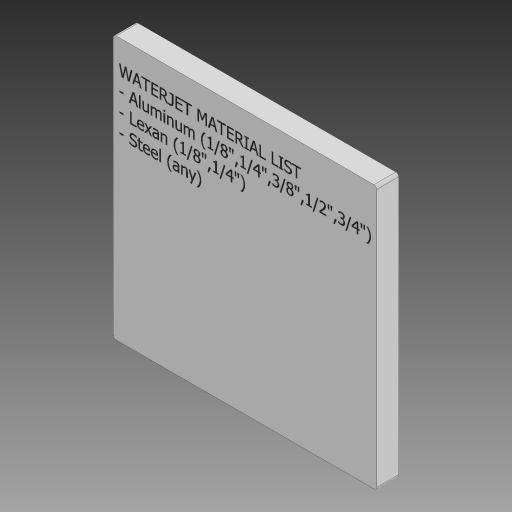
# Autodesk Inventor part: STOCK,WATERJET_MATERIALS
Saved by Autodesk Inventor 2023.4 (Build 274418000, 418)
## iProperties
Created: 2024-01-10
Part Number: STOCK,WATERJET_MATERIALS
Material: Generic
Document SubType Name: Modeling
Designer: dave.simone
Density: 1 g/cm^3
Appearance: Default
Author: dave.simone
Autodesk Inventor part; units mm, degrees
(part 1 of 2)
ref_plane "YZ Plane" through (0, 0, 0) normal (1, 0, 0) x (0, 1, 0)
ref_plane "XZ Plane" through (0, 0, 0) normal (0, 1, 0) x (-1, 0, 0)
ref_plane "XY Plane" through (0, 0, 0) normal (0, 0, 1) x (1, 0, 0)
sketch "Sketch1" plane through (0, 0, 0) normal (0, 0, 1) x (1, 0, 0)
  line L0 (-152.4, -152.4) -> (152.4, -152.4)
  line L1 (152.4, -152.4) -> (152.4, 152.4)
  line L2 (152.4, 152.4) -> (-152.4, 152.4)
  line L3 (-152.4, 152.4) -> (-152.4, -152.4)
  line L4 (-152.4, -152.4) -> (152.4, 152.4) construction
  line L5 (152.4, -152.4) -> (-152.4, 152.4) construction
  point P0 (0, 0)
  dimension "d0" = 304.8
  dimension "d1" = 304.8
  constraints: 12 end point, 2 midpoint, 2 parallel, 1 horizontal, 1 perpendicular
  measures "d0" distance of L1.end L2.end
  measures "d1" distance of L0.end L1.end
extrude "Extrusion1" add sketch "Sketch1" against normal blind 25.4
sketch "Sketch2" plane through (0, 0, 0) normal (0, 0, 1) x (1, 0, 0)
  line L0 (152.4, 152.4) -> (-152.4, 152.4) construction
  line L1 (-152.4, 152.4) -> (-152.4, -152.4) construction
  line L2 (-146.05, 127) -> (146.05, 127) construction
  line L3 (146.05, 127) -> (146.05, -127) construction
  line L4 (146.05, -127) -> (-146.05, -127) construction
  line L5 (-146.05, -127) -> (-146.05, 127) construction
  line L6 (-130.5301, 126.7736) -> (-133.7205, 114.0736)
  line L7 (-133.7205, 114.0736) -> (-135.6142, 114.0736)
  line L8 (-135.6142, 114.0736) -> (-138.1974, 124.6123)
  line L9 (-138.1974, 124.6123) -> (-140.7086, 114.0736)
  line L10 (-140.7086, 114.0736) -> (-142.5817, 114.0736)
  line L11 (-142.5817, 114.0736) -> (-145.8236, 126.7736)
  line L12 (-145.8236, 126.7736) -> (-144.0843, 126.7736)
  line L13 (-144.0843, 126.7736) -> (-141.5319, 116.2451)
  line L14 (-141.5319, 116.2451) -> (-139.0002, 126.7736)
  line L15 (-139.0002, 126.7736) -> (-137.2814, 126.7736)
  line L16 (-137.2814, 126.7736) -> (-134.7291, 116.1216)
  line L17 (-134.7291, 116.1216) -> (-132.187, 126.7736)
  line L18 (-132.187, 126.7736) -> (-130.5301, 126.7736)
  line L19 (-130.386, 114.0736) -> (-126.1046, 126.7736)
  line L20 (-126.1046, 126.7736) -> (-124.0257, 126.7736)
  line L21 (-124.0257, 126.7736) -> (-119.7443, 114.0736)
  line L22 (-119.7443, 114.0736) -> (-121.5248, 114.0736)
  line L23 (-121.5248, 114.0736) -> (-122.6775, 117.6242)
  line L24 (-122.6775, 117.6242) -> (-127.5249, 117.6242)
  line L25 (-127.5249, 117.6242) -> (-128.6776, 114.0736)
  line L26 (-128.6776, 114.0736) -> (-130.386, 114.0736)
  line L27 (-123.1406, 119.0651) -> (-125.1063, 125.0446)
  line L28 (-125.1063, 125.0446) -> (-127.0618, 119.0651)
  line L29 (-127.0618, 119.0651) -> (-123.1406, 119.0651)
  line L30 (-115.5762, 114.0736) -> (-115.5762, 125.271)
  line L31 (-115.5762, 125.271) -> (-119.837, 125.271)
  line L32 (-119.837, 125.271) -> (-119.837, 126.7736)
  line L33 (-119.837, 126.7736) -> (-109.6276, 126.7736)
  line L34 (-109.6276, 126.7736) -> (-109.6276, 125.271)
  line L35 (-109.6276, 125.271) -> (-113.8883, 125.271)
  line L36 (-113.8883, 125.271) -> (-113.8883, 114.0736)
  line L37 (-113.8883, 114.0736) -> (-115.5762, 114.0736)
  line L38 (-108.3411, 114.0736) -> (-108.3411, 126.7736)
  line L39 (-108.3411, 126.7736) -> (-100.3959, 126.7736)
  line L40 (-100.3959, 126.7736) -> (-100.3959, 125.271)
  line L41 (-100.3959, 125.271) -> (-106.6532, 125.271)
  line L42 (-106.6532, 125.271) -> (-106.6532, 121.7924)
  line L43 (-106.6532, 121.7924) -> (-100.8178, 121.7924)
  line L44 (-100.8178, 121.7924) -> (-100.8178, 120.2898)
  line L45 (-100.8178, 120.2898) -> (-106.6532, 120.2898)
  line L46 (-106.6532, 120.2898) -> (-106.6532, 115.5762)
  line L47 (-106.6532, 115.5762) -> (-100.3959, 115.5762)
  line L48 (-100.3959, 115.5762) -> (-100.3959, 114.0736)
  line L49 (-100.3959, 114.0736) -> (-108.3411, 114.0736)
  line L50 (-88.7147, 114.0736) -> (-90.9069, 114.0736)
  line L51 (-90.9069, 114.0736) -> (-94.9207, 119.1268)
  line L52 (-94.9207, 119.1268) -> (-96.8555, 119.1268)
  line L53 (-96.8555, 119.1268) -> (-96.8555, 114.0736)
  line L54 (-96.8555, 114.0736) -> (-98.5434, 114.0736)
  line L55 (-98.5434, 114.0736) -> (-98.5434, 126.7736)
  line L56 (-98.5434, 126.7736) -> (-95.2706, 126.7736)
  spline S0 degree 2 poles (-95.2706, 126.7736) (-94.1797, 126.7736) (-92.7079, 126.5369) (-92.039, 126.1046) knots 0 0 0 1 2 2 2
  spline S1 degree 2 poles (-92.039, 126.1046) (-91.37, 125.6724) (-90.5981, 124.3241) (-90.5981, 123.3259) knots 0 0 0 1 2 2 2
  spline S2 degree 2 poles (-90.5981, 123.3259) (-90.5981, 121.9365) (-92.0184, 120.0531) (-93.2328, 119.6002) knots 0 0 0 1 2 2 2
  line L57 (-93.2328, 119.6002) -> (-88.7147, 114.0736)
  spline S3 degree 2 poles (-92.358, 123.1921) (-92.358, 123.7478) (-92.7491, 124.602) (-93.1608, 124.8799) knots 0 0 0 1 2 2 2
  spline S4 degree 2 poles (-93.1608, 124.8799) (-93.521, 125.1166) (-94.4781, 125.3122) (-95.178, 125.3122) knots 0 0 0 1 2 2 2
  line L58 (-95.178, 125.3122) -> (-96.8555, 125.3122)
  line L59 (-96.8555, 125.3122) -> (-96.8555, 120.5368)
  line L60 (-96.8555, 120.5368) -> (-95.3735, 120.5368)
  spline S5 degree 2 poles (-95.3735, 120.5368) (-94.6428, 120.5368) (-93.4798, 120.7941) (-93.0784, 121.1955) knots 0 0 0 1 2 2 2
  spline S6 degree 2 poles (-93.0784, 121.1955) (-92.7079, 121.5454) (-92.358, 122.5334) (-92.358, 123.1921) knots 0 0 0 1 2 2 2
  spline S7 degree 2 poles (-82.9205, 117.3772) (-82.9205, 115.71) (-84.9583, 113.8986) (-86.677, 113.8986) knots 0 0 0 1 2 2 2
  spline S8 degree 2 poles (-86.677, 113.8986) (-87.0887, 113.8986) (-88.4575, 114.0427) (-88.9206, 114.1456) knots 0 0 0 1 2 2 2
  line L61 (-88.9206, 114.1456) -> (-88.9206, 115.7717)
  line L62 (-88.9206, 115.7717) -> (-88.828, 115.7717)
  spline S9 degree 2 poles (-88.828, 115.7717) (-88.478, 115.6482) (-87.4386, 115.36) (-86.9034, 115.36) knots 0 0 0 1 2 2 2
  spline S10 degree 2 poles (-86.9034, 115.36) (-86.1212, 115.36) (-85.1847, 115.7203) (-84.9686, 116.0496) knots 0 0 0 1 2 2 2
  spline S11 degree 2 poles (-84.9686, 116.0496) (-84.7318, 116.3892) (-84.6083, 117.3772) (-84.6083, 118.0256) knots 0 0 0 1 2 2 2
  line L63 (-84.6083, 118.0256) -> (-84.6083, 125.4254)
  line L64 (-84.6083, 125.4254) -> (-87.2945, 125.4254)
  line L65 (-87.2945, 125.4254) -> (-87.2945, 126.7736)
  line L66 (-87.2945, 126.7736) -> (-82.9205, 126.7736)
  line L67 (-82.9205, 126.7736) -> (-82.9205, 117.3772)
  line L68 (-80.4299, 114.0736) -> (-80.4299, 126.7736)
  line L69 (-80.4299, 126.7736) -> (-72.4847, 126.7736)
  line L70 (-72.4847, 126.7736) -> (-72.4847, 125.271)
  line L71 (-72.4847, 125.271) -> (-78.7421, 125.271)
  line L72 (-78.7421, 125.271) -> (-78.7421, 121.7924)
  line L73 (-78.7421, 121.7924) -> (-72.9066, 121.7924)
  line L74 (-72.9066, 121.7924) -> (-72.9066, 120.2898)
  line L75 (-72.9066, 120.2898) -> (-78.7421, 120.2898)
  line L76 (-78.7421, 120.2898) -> (-78.7421, 115.5762)
  line L77 (-78.7421, 115.5762) -> (-72.4847, 115.5762)
  line L78 (-72.4847, 115.5762) -> (-72.4847, 114.0736)
  line L79 (-72.4847, 114.0736) -> (-80.4299, 114.0736)
  line L80 (-67.6682, 114.0736) -> (-67.6682, 125.271)
  line L81 (-67.6682, 125.271) -> (-71.9289, 125.271)
  line L82 (-71.9289, 125.271) -> (-71.9289, 126.7736)
  line L83 (-71.9289, 126.7736) -> (-61.7195, 126.7736)
  line L84 (-61.7195, 126.7736) -> (-61.7195, 125.271)
  line L85 (-61.7195, 125.271) -> (-65.9803, 125.271)
  line L86 (-65.9803, 125.271) -> (-65.9803, 114.0736)
  line L87 (-65.9803, 114.0736) -> (-67.6682, 114.0736)
  line L88 (-44.0898, 114.0736) -> (-45.7776, 114.0736)
  line L89 (-45.7776, 114.0736) -> (-45.7776, 125.0137)
  line L90 (-45.7776, 125.0137) -> (-49.0916, 117.5728)
  line L91 (-49.0916, 117.5728) -> (-50.1207, 117.5728)
  line L92 (-50.1207, 117.5728) -> (-53.4038, 125.0137)
  line L93 (-53.4038, 125.0137) -> (-53.4038, 114.0736)
  line L94 (-53.4038, 114.0736) -> (-54.9784, 114.0736)
  line L95 (-54.9784, 114.0736) -> (-54.9784, 126.7736)
  line L96 (-54.9784, 126.7736) -> (-52.6731, 126.7736)
  line L97 (-52.6731, 126.7736) -> (-49.5032, 119.7032)
  line L98 (-49.5032, 119.7032) -> (-46.4363, 126.7736)
  line L99 (-46.4363, 126.7736) -> (-44.0898, 126.7736)
  line L100 (-44.0898, 126.7736) -> (-44.0898, 114.0736)
  line L101 (-42.8857, 114.0736) -> (-38.6043, 126.7736)
  line L102 (-38.6043, 126.7736) -> (-36.5254, 126.7736)
  line L103 (-36.5254, 126.7736) -> (-32.244, 114.0736)
  line L104 (-32.244, 114.0736) -> (-34.0245, 114.0736)
  line L105 (-34.0245, 114.0736) -> (-35.1771, 117.6242)
  line L106 (-35.1771, 117.6242) -> (-40.0246, 117.6242)
  line L107 (-40.0246, 117.6242) -> (-41.1772, 114.0736)
  line L108 (-41.1772, 114.0736) -> (-42.8857, 114.0736)
  line L109 (-35.6403, 119.0651) -> (-37.606, 125.0446)
  line L110 (-37.606, 125.0446) -> (-39.5614, 119.0651)
  line L111 (-39.5614, 119.0651) -> (-35.6403, 119.0651)
  line L112 (-28.0759, 114.0736) -> (-28.0759, 125.271)
  line L113 (-28.0759, 125.271) -> (-32.3366, 125.271)
  line L114 (-32.3366, 125.271) -> (-32.3366, 126.7736)
  line L115 (-32.3366, 126.7736) -> (-22.1272, 126.7736)
  line L116 (-22.1272, 126.7736) -> (-22.1272, 125.271)
  line L117 (-22.1272, 125.271) -> (-26.388, 125.271)
  line L118 (-26.388, 125.271) -> (-26.388, 114.0736)
  line L119 (-26.388, 114.0736) -> (-28.0759, 114.0736)
  line L120 (-20.8408, 114.0736) -> (-20.8408, 126.7736)
  line L121 (-20.8408, 126.7736) -> (-12.8955, 126.7736)
  line L122 (-12.8955, 126.7736) -> (-12.8955, 125.271)
  line L123 (-12.8955, 125.271) -> (-19.1529, 125.271)
  line L124 (-19.1529, 125.271) -> (-19.1529, 121.7924)
  line L125 (-19.1529, 121.7924) -> (-13.3175, 121.7924)
  line L126 (-13.3175, 121.7924) -> (-13.3175, 120.2898)
  line L127 (-13.3175, 120.2898) -> (-19.1529, 120.2898)
  line L128 (-19.1529, 120.2898) -> (-19.1529, 115.5762)
  line L129 (-19.1529, 115.5762) -> (-12.8955, 115.5762)
  line L130 (-12.8955, 115.5762) -> (-12.8955, 114.0736)
  line L131 (-12.8955, 114.0736) -> (-20.8408, 114.0736)
  line L132 (-1.2144, 114.0736) -> (-3.4066, 114.0736)
  line L133 (-3.4066, 114.0736) -> (-7.4203, 119.1268)
  line L134 (-7.4203, 119.1268) -> (-9.3552, 119.1268)
  line L135 (-9.3552, 119.1268) -> (-9.3552, 114.0736)
  line L136 (-9.3552, 114.0736) -> (-11.043, 114.0736)
  line L137 (-11.043, 114.0736) -> (-11.043, 126.7736)
  line L138 (-11.043, 126.7736) -> (-7.7703, 126.7736)
  spline S12 degree 2 poles (-7.7703, 126.7736) (-6.6793, 126.7736) (-5.2076, 126.5369) (-4.5387, 126.1046) knots 0 0 0 1 2 2 2
  spline S13 degree 2 poles (-4.5387, 126.1046) (-3.8697, 125.6724) (-3.0978, 124.3241) (-3.0978, 123.3259) knots 0 0 0 1 2 2 2
  spline S14 degree 2 poles (-3.0978, 123.3259) (-3.0978, 121.9365) (-4.5181, 120.0531) (-5.7325, 119.6002) knots 0 0 0 1 2 2 2
  line L139 (-5.7325, 119.6002) -> (-1.2144, 114.0736)
  spline S15 degree 2 poles (-4.8577, 123.1921) (-4.8577, 123.7478) (-5.2488, 124.602) (-5.6605, 124.8799) knots 0 0 0 1 2 2 2
  spline S16 degree 2 poles (-5.6605, 124.8799) (-6.0207, 125.1166) (-6.9778, 125.3122) (-7.6776, 125.3122) knots 0 0 0 1 2 2 2
  line L140 (-7.6776, 125.3122) -> (-9.3552, 125.3122)
  line L141 (-9.3552, 125.3122) -> (-9.3552, 120.5368)
  line L142 (-9.3552, 120.5368) -> (-7.8732, 120.5368)
  spline S17 degree 2 poles (-7.8732, 120.5368) (-7.1425, 120.5368) (-5.9795, 120.7941) (-5.5781, 121.1955) knots 0 0 0 1 2 2 2
  spline S18 degree 2 poles (-5.5781, 121.1955) (-5.2076, 121.5454) (-4.8577, 122.5334) (-4.8577, 123.1921) knots 0 0 0 1 2 2 2
  line L143 (4.2196, 114.0736) -> (-0.6998, 114.0736)
  line L144 (-0.6998, 114.0736) -> (-0.6998, 115.3703)
  line L145 (-0.6998, 115.3703) -> (0.916, 115.3703)
  line L146 (0.916, 115.3703) -> (0.916, 125.4768)
  line L147 (0.916, 125.4768) -> (-0.6998, 125.4768)
  line L148 (-0.6998, 125.4768) -> (-0.6998, 126.7736)
  line L149 (-0.6998, 126.7736) -> (4.2196, 126.7736)
  line L150 (4.2196, 126.7736) -> (4.2196, 125.4768)
  line L151 (4.2196, 125.4768) -> (2.6038, 125.4768)
  line L152 (2.6038, 125.4768) -> (2.6038, 115.3703)
  line L153 (2.6038, 115.3703) -> (4.2196, 115.3703)
  line L154 (4.2196, 115.3703) -> (4.2196, 114.0736)
  line L155 (4.94, 114.0736) -> (9.2214, 126.7736)
  line L156 (9.2214, 126.7736) -> (11.3003, 126.7736)
  line L157 (11.3003, 126.7736) -> (15.5817, 114.0736)
  line L158 (15.5817, 114.0736) -> (13.8012, 114.0736)
  line L159 (13.8012, 114.0736) -> (12.6485, 117.6242)
  line L160 (12.6485, 117.6242) -> (7.8011, 117.6242)
  line L161 (7.8011, 117.6242) -> (6.6485, 114.0736)
  line L162 (6.6485, 114.0736) -> (4.94, 114.0736)
  line L163 (12.1854, 119.0651) -> (10.2197, 125.0446)
  line L164 (10.2197, 125.0446) -> (8.2643, 119.0651)
  line L165 (8.2643, 119.0651) -> (12.1854, 119.0651)
  line L166 (24.1444, 114.0736) -> (16.7858, 114.0736)
  line L167 (16.7858, 114.0736) -> (16.7858, 126.7736)
  line L168 (16.7858, 126.7736) -> (18.4737, 126.7736)
  line L169 (18.4737, 126.7736) -> (18.4737, 115.5762)
  line L170 (18.4737, 115.5762) -> (24.1444, 115.5762)
  line L171 (24.1444, 115.5762) -> (24.1444, 114.0736)
  line L172 (38.2852, 114.0736) -> (30.9267, 114.0736)
  line L173 (30.9267, 114.0736) -> (30.9267, 126.7736)
  line L174 (30.9267, 126.7736) -> (32.6145, 126.7736)
  line L175 (32.6145, 126.7736) -> (32.6145, 115.5762)
  line L176 (32.6145, 115.5762) -> (38.2852, 115.5762)
  line L177 (38.2852, 115.5762) -> (38.2852, 114.0736)
  line L178 (44.0383, 114.0736) -> (39.1189, 114.0736)
  line L179 (39.1189, 114.0736) -> (39.1189, 115.3703)
  line L180 (39.1189, 115.3703) -> (40.7347, 115.3703)
  line L181 (40.7347, 115.3703) -> (40.7347, 125.4768)
  line L182 (40.7347, 125.4768) -> (39.1189, 125.4768)
  line L183 (39.1189, 125.4768) -> (39.1189, 126.7736)
  line L184 (39.1189, 126.7736) -> (44.0383, 126.7736)
  line L185 (44.0383, 126.7736) -> (44.0383, 125.4768)
  line L186 (44.0383, 125.4768) -> (42.4225, 125.4768)
  line L187 (42.4225, 125.4768) -> (42.4225, 115.3703)
  line L188 (42.4225, 115.3703) -> (44.0383, 115.3703)
  line L189 (44.0383, 115.3703) -> (44.0383, 114.0736)
  spline S19 degree 2 poles (49.6679, 113.8472) (48.2888, 113.8472) (46.354, 114.4235) (45.4998, 114.8352) knots 0 0 0 1 2 2 2
  line L190 (45.4998, 114.8352) -> (45.4998, 116.9553)
  line L191 (45.4998, 116.9553) -> (45.6233, 116.9553)
  spline S20 degree 2 poles (45.6233, 116.9553) (46.4569, 116.1731) (48.5667, 115.3086) (49.5444, 115.3086) knots 0 0 0 1 2 2 2
  spline S21 degree 2 poles (49.5444, 115.3086) (50.9441, 115.3086) (52.3746, 116.4716) (52.3746, 117.4287) knots 0 0 0 1 2 2 2
  spline S22 degree 2 poles (52.3746, 117.4287) (52.3746, 118.1903) (51.6233, 119.1371) (50.8103, 119.3738) knots 0 0 0 1 2 2 2
  spline S23 degree 2 poles (50.8103, 119.3738) (50.2237, 119.5385) (49.2459, 119.7649) (48.5152, 119.9502) knots 0 0 0 1 2 2 2
  spline S24 degree 2 poles (48.5152, 119.9502) (47.8566, 120.1251) (46.8171, 120.65) (46.4157, 121.072) knots 0 0 0 1 2 2 2
  spline S25 degree 2 poles (46.4157, 121.072) (46.0246, 121.4939) (45.5924, 122.626) (45.5924, 123.367) knots 0 0 0 1 2 2 2
  spline S26 degree 2 poles (45.5924, 123.367) (45.5924, 124.9108) (48.0006, 127) (49.8634, 127) knots 0 0 0 1 2 2 2
  spline S27 degree 2 poles (49.8634, 127) (50.9338, 127) (52.8275, 126.578) (53.6405, 126.1767) knots 0 0 0 1 2 2 2
  line L192 (53.6405, 126.1767) -> (53.6405, 124.1595)
  line L193 (53.6405, 124.1595) -> (53.517, 124.1595)
  spline S28 degree 2 poles (53.517, 124.1595) (52.9098, 124.7152) (51.0161, 125.5386) (49.9767, 125.5386) knots 0 0 0 1 2 2 2
  spline S29 degree 2 poles (49.9767, 125.5386) (48.8034, 125.5386) (47.3523, 124.4374) (47.3523, 123.542) knots 0 0 0 1 2 2 2
  spline S30 degree 2 poles (47.3523, 123.542) (47.3523, 122.7392) (48.2065, 121.7821) (49.0092, 121.566) knots 0 0 0 1 2 2 2
  spline S31 degree 2 poles (49.0092, 121.566) (49.5444, 121.4219) (51.0985, 121.0514) (51.613, 120.897) knots 0 0 0 1 2 2 2
  spline S32 degree 2 poles (51.613, 120.897) (52.9201, 120.4956) (54.1345, 118.8798) (54.1345, 117.6963) knots 0 0 0 1 2 2 2
  spline S33 degree 2 poles (54.1345, 117.6963) (54.1345, 116.945) (53.5273, 115.5041) (52.9818, 114.9998) knots 0 0 0 1 2 2 2
  spline S34 degree 2 poles (52.9818, 114.9998) (52.3746, 114.4441) (50.8309, 113.8472) (49.6679, 113.8472) knots 0 0 0 1 2 2 2
  line L194 (58.8173, 114.0736) -> (58.8173, 125.271)
  line L195 (58.8173, 125.271) -> (54.5565, 125.271)
  line L196 (54.5565, 125.271) -> (54.5565, 126.7736)
  line L197 (54.5565, 126.7736) -> (64.7659, 126.7736)
  line L198 (64.7659, 126.7736) -> (64.7659, 125.271)
  line L199 (64.7659, 125.271) -> (60.5051, 125.271)
  line L200 (60.5051, 125.271) -> (60.5051, 114.0736)
  line L201 (60.5051, 114.0736) -> (58.8173, 114.0736)
  line L202 (-140.4719, 97.949) -> (-145.2781, 97.949)
  line L203 (-145.2781, 97.949) -> (-145.2781, 99.4928)
  line L204 (-145.2781, 99.4928) -> (-140.4719, 99.4928)
  line L205 (-140.4719, 99.4928) -> (-140.4719, 97.949)
  line L206 (-134.338, 93.1634) -> (-130.0566, 105.8634)
  line L207 (-130.0566, 105.8634) -> (-127.9777, 105.8634)
  line L208 (-127.9777, 105.8634) -> (-123.6964, 93.1634)
  line L209 (-123.6964, 93.1634) -> (-125.4768, 93.1634)
  line L210 (-125.4768, 93.1634) -> (-126.6295, 96.714)
  line L211 (-126.6295, 96.714) -> (-131.4769, 96.714)
  line L212 (-131.4769, 96.714) -> (-132.6296, 93.1634)
  line L213 (-132.6296, 93.1634) -> (-134.338, 93.1634)
  line L214 (-127.0926, 98.1549) -> (-129.0583, 104.1344)
  line L215 (-129.0583, 104.1344) -> (-131.0138, 98.1549)
  line L216 (-131.0138, 98.1549) -> (-127.0926, 98.1549)
  line L217 (-120.9793, 93.1634) -> (-122.5848, 93.1634)
  line L218 (-122.5848, 93.1634) -> (-122.5848, 106.4294)
  line L219 (-122.5848, 106.4294) -> (-120.9793, 106.4294)
  line L220 (-120.9793, 106.4294) -> (-120.9793, 93.1634)
  line L221 (-111.2125, 93.1634) -> (-112.818, 93.1634)
  line L222 (-112.818, 93.1634) -> (-112.818, 94.2131)
  spline S35 degree 2 poles (-112.818, 94.2131) (-113.559, 93.5647) (-114.8866, 92.8958) (-115.71, 92.8958) knots 0 0 0 1 2 2 2
  spline S36 degree 2 poles (-115.71, 92.8958) (-116.3275, 92.8958) (-117.4287, 93.3075) (-117.8301, 93.75) knots 0 0 0 1 2 2 2
  spline S37 degree 2 poles (-117.8301, 93.75) (-118.2417, 94.1925) (-118.6946, 95.5408) (-118.6946, 96.5082) knots 0 0 0 1 2 2 2
  line L223 (-118.6946, 96.5082) -> (-118.6946, 102.6935)
  line L224 (-118.6946, 102.6935) -> (-117.0891, 102.6935)
  line L225 (-117.0891, 102.6935) -> (-117.0891, 97.2595)
  spline S38 degree 2 poles (-117.0891, 97.2595) (-117.0891, 96.4979) (-116.9759, 95.4996) (-116.7803, 95.1291) knots 0 0 0 1 2 2 2
  spline S39 degree 2 poles (-116.7803, 95.1291) (-116.5848, 94.7586) (-115.9158, 94.419) (-115.288, 94.419) knots 0 0 0 1 2 2 2
  spline S40 degree 2 poles (-115.288, 94.419) (-114.7014, 94.419) (-113.3737, 95.0879) (-112.818, 95.5716) knots 0 0 0 1 2 2 2
  line L226 (-112.818, 95.5716) -> (-112.818, 102.6935)
  line L227 (-112.818, 102.6935) -> (-111.2125, 102.6935)
  line L228 (-111.2125, 102.6935) -> (-111.2125, 93.1634)
  line L229 (-98.0802, 93.1634) -> (-98.0802, 98.6797)
  spline S41 degree 2 poles (-98.0802, 98.6797) (-98.0802, 99.3384) (-98.1831, 100.4602) (-98.3478, 100.769) knots 0 0 0 1 2 2 2
  spline S42 degree 2 poles (-98.3478, 100.769) (-98.5125, 101.1086) (-99.1403, 101.4379) (-99.6857, 101.4379) knots 0 0 0 1 2 2 2
  spline S43 degree 2 poles (-99.6857, 101.4379) (-100.1797, 101.4379) (-101.3118, 100.8307) (-101.9088, 100.2544) knots 0 0 0 1 2 2 2
  spline S44 degree 2 poles (-101.9088, 100.2544) (-101.8985, 100.1103) (-101.8779, 99.7089) (-101.8779, 99.4413) knots 0 0 0 1 2 2 2
  line L230 (-101.8779, 99.4413) -> (-101.8779, 93.1634)
  line L231 (-101.8779, 93.1634) -> (-103.4834, 93.1634)
  line L232 (-103.4834, 93.1634) -> (-103.4834, 98.6797)
  spline S45 degree 2 poles (-103.4834, 98.6797) (-103.4834, 99.3384) (-103.5863, 100.4602) (-103.751, 100.769) knots 0 0 0 1 2 2 2
  spline S46 degree 2 poles (-103.751, 100.769) (-103.9156, 101.1086) (-104.5434, 101.4379) (-105.0889, 101.4379) knots 0 0 0 1 2 2 2
  spline S47 degree 2 poles (-105.0889, 101.4379) (-105.6035, 101.4379) (-106.7459, 100.7895) (-107.281, 100.2852) knots 0 0 0 1 2 2 2
  line L233 (-107.281, 100.2852) -> (-107.281, 93.1634)
  line L234 (-107.281, 93.1634) -> (-108.8865, 93.1634)
  line L235 (-108.8865, 93.1634) -> (-108.8865, 102.6935)
  line L236 (-108.8865, 102.6935) -> (-107.281, 102.6935)
  line L237 (-107.281, 102.6935) -> (-107.281, 101.6438)
  spline S48 degree 2 poles (-107.281, 101.6438) (-106.6532, 102.2716) (-105.4182, 102.9611) (-104.6772, 102.9611) knots 0 0 0 1 2 2 2
  spline S49 degree 2 poles (-104.6772, 102.9611) (-103.8333, 102.9611) (-102.5263, 102.1892) (-102.1866, 101.3144) knots 0 0 0 1 2 2 2
  spline S50 degree 2 poles (-102.1866, 101.3144) (-101.4559, 102.1275) (-100.0768, 102.9611) (-99.2741, 102.9611) knots 0 0 0 1 2 2 2
  spline S51 degree 2 poles (-99.2741, 102.9611) (-98.6566, 102.9611) (-97.648, 102.5803) (-97.2775, 102.1481) knots 0 0 0 1 2 2 2
  spline S52 degree 2 poles (-97.2775, 102.1481) (-96.8967, 101.7158) (-96.4747, 100.419) (-96.4747, 99.4413) knots 0 0 0 1 2 2 2
  line L238 (-96.4747, 99.4413) -> (-96.4747, 93.1634)
  line L239 (-96.4747, 93.1634) -> (-98.0802, 93.1634)
  line L240 (-92.5844, 93.1634) -> (-94.19, 93.1634)
  line L241 (-94.19, 93.1634) -> (-94.19, 102.6935)
  line L242 (-94.19, 102.6935) -> (-92.5844, 102.6935)
  line L243 (-92.5844, 102.6935) -> (-92.5844, 93.1634)
  line L244 (-92.4712, 104.2784) -> (-94.2929, 104.2784)
  line L245 (-94.2929, 104.2784) -> (-94.2929, 105.9457)
  line L246 (-94.2929, 105.9457) -> (-92.4712, 105.9457)
  line L247 (-92.4712, 105.9457) -> (-92.4712, 104.2784)
  line L248 (-82.7455, 93.1634) -> (-84.3511, 93.1634)
  line L249 (-84.3511, 93.1634) -> (-84.3511, 98.5974)
  spline S53 degree 2 poles (-84.3511, 98.5974) (-84.3511, 99.2561) (-84.4746, 100.3882) (-84.6598, 100.7278) knots 0 0 0 1 2 2 2
  spline S54 degree 2 poles (-84.6598, 100.7278) (-84.8553, 101.088) (-85.5552, 101.4379) (-86.1521, 101.4379) knots 0 0 0 1 2 2 2
  spline S55 degree 2 poles (-86.1521, 101.4379) (-86.749, 101.4379) (-88.0149, 100.7998) (-88.6221, 100.2852) knots 0 0 0 1 2 2 2
  line L250 (-88.6221, 100.2852) -> (-88.6221, 93.1634)
  line L251 (-88.6221, 93.1634) -> (-90.2276, 93.1634)
  line L252 (-90.2276, 93.1634) -> (-90.2276, 102.6935)
  line L253 (-90.2276, 102.6935) -> (-88.6221, 102.6935)
  line L254 (-88.6221, 102.6935) -> (-88.6221, 101.6335)
  spline S56 degree 2 poles (-88.6221, 101.6335) (-87.9017, 102.2818) (-86.5123, 102.9611) (-85.7301, 102.9611) knots 0 0 0 1 2 2 2
  spline S57 degree 2 poles (-85.7301, 102.9611) (-84.3305, 102.9611) (-82.7455, 101.1086) (-82.7455, 99.3487) knots 0 0 0 1 2 2 2
  line L255 (-82.7455, 99.3487) -> (-82.7455, 93.1634)
  line L256 (-73.0816, 93.1634) -> (-74.6871, 93.1634)
  line L257 (-74.6871, 93.1634) -> (-74.6871, 94.2131)
  spline S58 degree 2 poles (-74.6871, 94.2131) (-75.4281, 93.5647) (-76.7558, 92.8958) (-77.5791, 92.8958) knots 0 0 0 1 2 2 2
  spline S59 degree 2 poles (-77.5791, 92.8958) (-78.1966, 92.8958) (-79.2978, 93.3075) (-79.6992, 93.75) knots 0 0 0 1 2 2 2
  spline S60 degree 2 poles (-79.6992, 93.75) (-80.1109, 94.1925) (-80.5637, 95.5408) (-80.5637, 96.5082) knots 0 0 0 1 2 2 2
  line L258 (-80.5637, 96.5082) -> (-80.5637, 102.6935)
  line L259 (-80.5637, 102.6935) -> (-78.9582, 102.6935)
  line L260 (-78.9582, 102.6935) -> (-78.9582, 97.2595)
  spline S61 degree 2 poles (-78.9582, 97.2595) (-78.9582, 96.4979) (-78.845, 95.4996) (-78.6494, 95.1291) knots 0 0 0 1 2 2 2
  spline S62 degree 2 poles (-78.6494, 95.1291) (-78.4539, 94.7586) (-77.7849, 94.419) (-77.1571, 94.419) knots 0 0 0 1 2 2 2
  spline S63 degree 2 poles (-77.1571, 94.419) (-76.5705, 94.419) (-75.2429, 95.0879) (-74.6871, 95.5716) knots 0 0 0 1 2 2 2
  line L261 (-74.6871, 95.5716) -> (-74.6871, 102.6935)
  line L262 (-74.6871, 102.6935) -> (-73.0816, 102.6935)
  line L263 (-73.0816, 102.6935) -> (-73.0816, 93.1634)
  line L264 (-59.9494, 93.1634) -> (-59.9494, 98.6797)
  spline S64 degree 2 poles (-59.9494, 98.6797) (-59.9494, 99.3384) (-60.0523, 100.4602) (-60.2169, 100.769) knots 0 0 0 1 2 2 2
  spline S65 degree 2 poles (-60.2169, 100.769) (-60.3816, 101.1086) (-61.0094, 101.4379) (-61.5549, 101.4379) knots 0 0 0 1 2 2 2
  spline S66 degree 2 poles (-61.5549, 101.4379) (-62.0489, 101.4379) (-63.181, 100.8307) (-63.7779, 100.2544) knots 0 0 0 1 2 2 2
  spline S67 degree 2 poles (-63.7779, 100.2544) (-63.7676, 100.1103) (-63.747, 99.7089) (-63.747, 99.4413) knots 0 0 0 1 2 2 2
  line L265 (-63.747, 99.4413) -> (-63.747, 93.1634)
  line L266 (-63.747, 93.1634) -> (-65.3525, 93.1634)
  line L267 (-65.3525, 93.1634) -> (-65.3525, 98.6797)
  spline S68 degree 2 poles (-65.3525, 98.6797) (-65.3525, 99.3384) (-65.4554, 100.4602) (-65.6201, 100.769) knots 0 0 0 1 2 2 2
  spline S69 degree 2 poles (-65.6201, 100.769) (-65.7848, 101.1086) (-66.4126, 101.4379) (-66.958, 101.4379) knots 0 0 0 1 2 2 2
  spline S70 degree 2 poles (-66.958, 101.4379) (-67.4726, 101.4379) (-68.615, 100.7895) (-69.1502, 100.2852) knots 0 0 0 1 2 2 2
  line L268 (-69.1502, 100.2852) -> (-69.1502, 93.1634)
  line L269 (-69.1502, 93.1634) -> (-70.7557, 93.1634)
  line L270 (-70.7557, 93.1634) -> (-70.7557, 102.6935)
  line L271 (-70.7557, 102.6935) -> (-69.1502, 102.6935)
  line L272 (-69.1502, 102.6935) -> (-69.1502, 101.6438)
  spline S71 degree 2 poles (-69.1502, 101.6438) (-68.5224, 102.2716) (-67.2874, 102.9611) (-66.5464, 102.9611) knots 0 0 0 1 2 2 2
  spline S72 degree 2 poles (-66.5464, 102.9611) (-65.7024, 102.9611) (-64.3954, 102.1892) (-64.0558, 101.3144) knots 0 0 0 1 2 2 2
  spline S73 degree 2 poles (-64.0558, 101.3144) (-63.325, 102.1275) (-61.9459, 102.9611) (-61.1432, 102.9611) knots 0 0 0 1 2 2 2
  spline S74 degree 2 poles (-61.1432, 102.9611) (-60.5257, 102.9611) (-59.5171, 102.5803) (-59.1466, 102.1481) knots 0 0 0 1 2 2 2
  spline S75 degree 2 poles (-59.1466, 102.1481) (-58.7658, 101.7158) (-58.3438, 100.419) (-58.3438, 99.4413) knots 0 0 0 1 2 2 2
  line L273 (-58.3438, 99.4413) -> (-58.3438, 93.1634)
  line L274 (-58.3438, 93.1634) -> (-59.9494, 93.1634)
  line L275 (-45.7468, 89.6539) -> (-47.7022, 89.6539)
  spline S76 degree 2 poles (-47.7022, 89.6539) (-49.1842, 91.4138) (-50.8823, 95.3555) (-50.8823, 98.0416) knots 0 0 0 1 2 2 2
  spline S77 degree 2 poles (-50.8823, 98.0416) (-50.8823, 100.666) (-49.2048, 104.6695) (-47.7022, 106.4294) knots 0 0 0 1 2 2 2
  line L276 (-47.7022, 106.4294) -> (-45.7468, 106.4294)
  line L277 (-45.7468, 106.4294) -> (-45.7468, 106.3471)
  spline S78 degree 2 poles (-45.7468, 106.3471) (-46.4363, 105.7193) (-47.6919, 104.0932) (-48.2271, 103.0126) knots 0 0 0 1 2 2 2
  spline S79 degree 2 poles (-48.2271, 103.0126) (-48.7417, 101.9628) (-49.3797, 99.4413) (-49.3797, 98.0416) knots 0 0 0 1 2 2 2
  spline S80 degree 2 poles (-49.3797, 98.0416) (-49.3797, 96.5802) (-48.7622, 94.1617) (-48.2271, 93.0707) knots 0 0 0 1 2 2 2
  spline S81 degree 2 poles (-48.2271, 93.0707) (-47.7125, 92.021) (-46.4054, 90.3228) (-45.7468, 89.7362) knots 0 0 0 1 2 2 2
  line L278 (-45.7468, 89.7362) -> (-45.7468, 89.6539)
  line L279 (-36.9885, 93.1634) -> (-43.1841, 93.1634)
  line L280 (-43.1841, 93.1634) -> (-43.1841, 94.4601)
  line L281 (-43.1841, 94.4601) -> (-40.8788, 94.4601)
  line L282 (-40.8788, 94.4601) -> (-40.8788, 102.9714)
  line L283 (-40.8788, 102.9714) -> (-43.1841, 102.9714)
  line L284 (-43.1841, 102.9714) -> (-43.1841, 104.1344)
  spline S82 degree 2 poles (-43.1841, 104.1344) (-41.8771, 104.1344) (-40.6421, 104.8754) (-40.5597, 105.9045) knots 0 0 0 1 2 2 2
  line L285 (-40.5597, 105.9045) -> (-39.2424, 105.9045)
  line L286 (-39.2424, 105.9045) -> (-39.2424, 94.4601)
  line L287 (-39.2424, 94.4601) -> (-36.9885, 94.4601)
  line L288 (-36.9885, 94.4601) -> (-36.9885, 93.1634)
  line L289 (-29.3726, 106.4294) -> (-34.3435, 90.4052)
  line L290 (-34.3435, 90.4052) -> (-35.7844, 90.4052)
  line L291 (-35.7844, 90.4052) -> (-30.834, 106.4294)
  line L292 (-30.834, 106.4294) -> (-29.3726, 106.4294)
  spline S83 degree 2 poles (-24.1341, 92.8752) (-25.081, 92.8752) (-26.635, 93.4412) (-27.1805, 93.9661) knots 0 0 0 1 2 2 2
  spline S84 degree 2 poles (-27.1805, 93.9661) (-27.7156, 94.4807) (-28.2714, 95.8804) (-28.2714, 96.6728) knots 0 0 0 1 2 2 2
  spline S85 degree 2 poles (-28.2714, 96.6728) (-28.2714, 97.702) (-27.1702, 99.431) (-26.1204, 99.9456) knots 0 0 0 1 2 2 2
  line L293 (-26.1204, 99.9456) -> (-26.1204, 99.9971)
  spline S86 degree 2 poles (-26.1204, 99.9971) (-27.057, 100.5425) (-27.9626, 101.8393) (-27.9626, 102.8067) knots 0 0 0 1 2 2 2
  spline S87 degree 2 poles (-27.9626, 102.8067) (-27.9626, 104.2373) (-25.8014, 106.1515) (-24.1341, 106.1515) knots 0 0 0 1 2 2 2
  spline S88 degree 2 poles (-24.1341, 106.1515) (-22.4051, 106.1515) (-20.3159, 104.3402) (-20.3159, 102.9199) knots 0 0 0 1 2 2 2
  spline S89 degree 2 poles (-20.3159, 102.9199) (-20.3159, 102.0657) (-21.3142, 100.3985) (-22.2507, 99.925) knots 0 0 0 1 2 2 2
  line L294 (-22.2507, 99.925) -> (-22.2507, 99.8736)
  spline S90 degree 2 poles (-22.2507, 99.8736) (-21.1392, 99.359) (-19.9968, 97.877) (-19.9968, 96.7037) knots 0 0 0 1 2 2 2
  spline S91 degree 2 poles (-19.9968, 96.7037) (-19.9968, 95.0776) (-22.3639, 92.8752) (-24.1341, 92.8752) knots 0 0 0 1 2 2 2
  spline S92 degree 2 poles (-21.7464, 96.5391) (-21.7464, 97.3212) (-22.3639, 98.2475) (-23.2387, 98.7209) knots 0 0 0 1 2 2 2
  spline S93 degree 2 poles (-23.2387, 98.7209) (-23.5269, 98.8856) (-24.4943, 99.2664) (-25.1015, 99.5134) knots 0 0 0 1 2 2 2
  spline S94 degree 2 poles (-25.1015, 99.5134) (-25.8014, 99.0502) (-26.5527, 97.6711) (-26.5527, 96.7963) knots 0 0 0 1 2 2 2
  spline S95 degree 2 poles (-26.5527, 96.7963) (-26.5527, 95.6437) (-25.1633, 94.1411) (-24.1135, 94.1411) knots 0 0 0 1 2 2 2
  spline S96 degree 2 poles (-24.1135, 94.1411) (-23.0432, 94.1411) (-21.7464, 95.4275) (-21.7464, 96.5391) knots 0 0 0 1 2 2 2
  spline S97 degree 2 poles (-21.9831, 102.8993) (-21.9831, 103.7536) (-23.1255, 104.8959) (-24.1444, 104.8959) knots 0 0 0 1 2 2 2
  spline S98 degree 2 poles (-24.1444, 104.8959) (-25.0707, 104.8959) (-26.2542, 103.8771) (-26.2542, 103.0023) knots 0 0 0 1 2 2 2
  spline S99 degree 2 poles (-26.2542, 103.0023) (-26.2542, 102.3745) (-25.647, 101.4997) (-25.0398, 101.1498) knots 0 0 0 1 2 2 2
  spline S100 degree 2 poles (-25.0398, 101.1498) (-24.7825, 101.0057) (-23.6916, 100.5014) (-23.249, 100.3573) knots 0 0 0 1 2 2 2
  spline S101 degree 2 poles (-23.249, 100.3573) (-22.508, 100.9233) (-21.9831, 102.1275) (-21.9831, 102.8993) knots 0 0 0 1 2 2 2
  line L295 (-16.5388, 106.4294) -> (-16.9093, 101.4894)
  line L296 (-16.9093, 101.4894) -> (-18.0311, 101.4894)
  line L297 (-18.0311, 101.4894) -> (-18.4016, 106.4294)
  line L298 (-18.4016, 106.4294) -> (-16.5388, 106.4294)
  line L299 (-13.3278, 106.4294) -> (-13.6983, 101.4894)
  line L300 (-13.6983, 101.4894) -> (-14.8201, 101.4894)
  line L301 (-14.8201, 101.4894) -> (-15.1906, 106.4294)
  line L302 (-15.1906, 106.4294) -> (-13.3278, 106.4294)
  line L303 (-8.0996, 95.5922) -> (-10.4873, 90.0038)
  line L304 (-10.4873, 90.0038) -> (-11.7326, 90.0038)
  line L305 (-11.7326, 90.0038) -> (-10.23, 95.5922)
  line L306 (-10.23, 95.5922) -> (-8.0996, 95.5922)
  line L307 (1.0498, 93.1634) -> (-5.1459, 93.1634)
  line L308 (-5.1459, 93.1634) -> (-5.1459, 94.4601)
  line L309 (-5.1459, 94.4601) -> (-2.8405, 94.4601)
  line L310 (-2.8405, 94.4601) -> (-2.8405, 102.9714)
  line L311 (-2.8405, 102.9714) -> (-5.1459, 102.9714)
  line L312 (-5.1459, 102.9714) -> (-5.1459, 104.1344)
  spline S102 degree 2 poles (-5.1459, 104.1344) (-3.8388, 104.1344) (-2.6038, 104.8754) (-2.5215, 105.9045) knots 0 0 0 1 2 2 2
  line L313 (-2.5215, 105.9045) -> (-1.2041, 105.9045)
  line L314 (-1.2041, 105.9045) -> (-1.2041, 94.4601)
  line L315 (-1.2041, 94.4601) -> (1.0498, 94.4601)
  line L316 (1.0498, 94.4601) -> (1.0498, 93.1634)
  line L317 (8.6656, 106.4294) -> (3.6947, 90.4052)
  line L318 (3.6947, 90.4052) -> (2.2539, 90.4052)
  line L319 (2.2539, 90.4052) -> (7.2042, 106.4294)
  line L320 (7.2042, 106.4294) -> (8.6656, 106.4294)
  line L321 (18.237, 97.5271) -> (16.7241, 97.5271)
  line L322 (16.7241, 97.5271) -> (16.7241, 93.1634)
  line L323 (16.7241, 93.1634) -> (15.0877, 93.1634)
  line L324 (15.0877, 93.1634) -> (15.0877, 97.5271)
  line L325 (15.0877, 97.5271) -> (9.4787, 97.5271)
  line L326 (9.4787, 97.5271) -> (9.4787, 99.3178)
  line L327 (9.4787, 99.3178) -> (15.1597, 105.8634)
  line L328 (15.1597, 105.8634) -> (16.7241, 105.8634)
  line L329 (16.7241, 105.8634) -> (16.7241, 98.8959)
  line L330 (16.7241, 98.8959) -> (18.237, 98.8959)
  line L331 (18.237, 98.8959) -> (18.237, 97.5271)
  line L332 (15.0877, 98.8959) -> (15.0877, 103.8565)
  line L333 (15.0877, 103.8565) -> (10.8166, 98.8959)
  line L334 (10.8166, 98.8959) -> (15.0877, 98.8959)
  line L335 (24.7105, 106.4294) -> (24.3399, 101.4894)
  line L336 (24.3399, 101.4894) -> (23.2181, 101.4894)
  line L337 (23.2181, 101.4894) -> (22.8476, 106.4294)
  line L338 (22.8476, 106.4294) -> (24.7105, 106.4294)
  line L339 (21.4994, 106.4294) -> (21.1289, 101.4894)
  line L340 (21.1289, 101.4894) -> (20.0071, 101.4894)
  line L341 (20.0071, 101.4894) -> (19.6366, 106.4294)
  line L342 (19.6366, 106.4294) -> (21.4994, 106.4294)
  line L343 (29.9387, 95.5922) -> (27.551, 90.0038)
  line L344 (27.551, 90.0038) -> (26.3057, 90.0038)
  line L345 (26.3057, 90.0038) -> (27.8083, 95.5922)
  line L346 (27.8083, 95.5922) -> (29.9387, 95.5922)
  spline S103 degree 2 poles (35.3212, 104.6592) (34.8581, 104.6592) (33.9421, 104.4328) (33.4996, 104.2579) knots 0 0 0 1 2 2 2
  spline S104 degree 2 poles (33.4996, 104.2579) (33.0879, 104.0829) (32.4807, 103.7124) (32.244, 103.5477) knots 0 0 0 1 2 2 2
  line L347 (32.244, 103.5477) -> (32.1411, 103.5477)
  line L348 (32.1411, 103.5477) -> (32.1411, 105.3488)
  spline S105 degree 2 poles (32.1411, 105.3488) (32.6968, 105.6472) (34.6008, 106.131) (35.455, 106.131) knots 0 0 0 1 2 2 2
  spline S106 degree 2 poles (35.455, 106.131) (36.3195, 106.131) (37.606, 105.781) (38.1309, 105.4105) knots 0 0 0 1 2 2 2
  spline S107 degree 2 poles (38.1309, 105.4105) (38.6866, 105.0092) (39.263, 103.8462) (39.263, 103.064) knots 0 0 0 1 2 2 2
  spline S108 degree 2 poles (39.263, 103.064) (39.263, 102.0143) (37.8839, 100.4293) (36.9164, 100.2235) knots 0 0 0 1 2 2 2
  line L349 (36.9164, 100.2235) -> (36.9164, 100.1)
  spline S109 degree 2 poles (36.9164, 100.1) (37.3178, 100.0177) (38.2338, 99.6472) (38.6249, 99.2767) knots 0 0 0 1 2 2 2
  spline S110 degree 2 poles (38.6249, 99.2767) (39.016, 98.9164) (39.51, 97.7638) (39.51, 96.9301) knots 0 0 0 1 2 2 2
  spline S111 degree 2 poles (39.51, 96.9301) (39.51, 96.0759) (38.9233, 94.6248) (38.3882, 94.069) knots 0 0 0 1 2 2 2
  spline S112 degree 2 poles (38.3882, 94.069) (37.8324, 93.4927) (36.2578, 92.8958) (35.2595, 92.8958) knots 0 0 0 1 2 2 2
  spline S113 degree 2 poles (35.2595, 92.8958) (34.3023, 92.8958) (32.4293, 93.3589) (31.7912, 93.678) knots 0 0 0 1 2 2 2
  line L350 (31.7912, 93.678) -> (31.7912, 95.479)
  line L351 (31.7912, 95.479) -> (31.9147, 95.479)
  spline S114 degree 2 poles (31.9147, 95.479) (32.4498, 95.0879) (34.2612, 94.3675) (35.1566, 94.3675) knots 0 0 0 1 2 2 2
  spline S115 degree 2 poles (35.1566, 94.3675) (35.6814, 94.3675) (36.7312, 94.6968) (37.0811, 95.0776) knots 0 0 0 1 2 2 2
  spline S116 degree 2 poles (37.0811, 95.0776) (37.4207, 95.4584) (37.781, 96.3641) (37.781, 97.0536) knots 0 0 0 1 2 2 2
  spline S117 degree 2 poles (37.781, 97.0536) (37.781, 97.7432) (37.3796, 98.6386) (37.0194, 98.8959) knots 0 0 0 1 2 2 2
  spline S118 degree 2 poles (37.0194, 98.8959) (36.6592, 99.1532) (35.6814, 99.3487) (35.1051, 99.3487) knots 0 0 0 1 2 2 2
  line L352 (35.1051, 99.3487) -> (34.3847, 99.3487)
  line L353 (34.3847, 99.3487) -> (34.3847, 100.7587)
  line L354 (34.3847, 100.7587) -> (34.9507, 100.7587)
  spline S119 degree 2 poles (34.9507, 100.7587) (36.0931, 100.7587) (37.534, 101.8496) (37.534, 102.8891) knots 0 0 0 1 2 2 2
  spline S120 degree 2 poles (37.534, 102.8891) (37.534, 103.3728) (37.1634, 104.0623) (36.865, 104.2681) knots 0 0 0 1 2 2 2
  spline S121 degree 2 poles (36.865, 104.2681) (36.5459, 104.4843) (35.7638, 104.6592) (35.3212, 104.6592) knots 0 0 0 1 2 2 2
  line L355 (46.7039, 106.4294) -> (41.733, 90.4052)
  line L356 (41.733, 90.4052) -> (40.2921, 90.4052)
  line L357 (40.2921, 90.4052) -> (45.2425, 106.4294)
  line L358 (45.2425, 106.4294) -> (46.7039, 106.4294)
  spline S122 degree 2 poles (51.9424, 92.8752) (50.9955, 92.8752) (49.4415, 93.4412) (48.896, 93.9661) knots 0 0 0 1 2 2 2
  spline S123 degree 2 poles (48.896, 93.9661) (48.3609, 94.4807) (47.8051, 95.8804) (47.8051, 96.6728) knots 0 0 0 1 2 2 2
  spline S124 degree 2 poles (47.8051, 96.6728) (47.8051, 97.702) (48.9063, 99.431) (49.9561, 99.9456) knots 0 0 0 1 2 2 2
  line L359 (49.9561, 99.9456) -> (49.9561, 99.9971)
  spline S125 degree 2 poles (49.9561, 99.9971) (49.0195, 100.5425) (48.1139, 101.8393) (48.1139, 102.8067) knots 0 0 0 1 2 2 2
  spline S126 degree 2 poles (48.1139, 102.8067) (48.1139, 104.2373) (50.2751, 106.1515) (51.9424, 106.1515) knots 0 0 0 1 2 2 2
  spline S127 degree 2 poles (51.9424, 106.1515) (53.6714, 106.1515) (55.7606, 104.3402) (55.7606, 102.9199) knots 0 0 0 1 2 2 2
  spline S128 degree 2 poles (55.7606, 102.9199) (55.7606, 102.0657) (54.7623, 100.3985) (53.8258, 99.925) knots 0 0 0 1 2 2 2
  line L360 (53.8258, 99.925) -> (53.8258, 99.8736)
  spline S129 degree 2 poles (53.8258, 99.8736) (54.9373, 99.359) (56.0797, 97.877) (56.0797, 96.7037) knots 0 0 0 1 2 2 2
  spline S130 degree 2 poles (56.0797, 96.7037) (56.0797, 95.0776) (53.7126, 92.8752) (51.9424, 92.8752) knots 0 0 0 1 2 2 2
  spline S131 degree 2 poles (54.3301, 96.5391) (54.3301, 97.3212) (53.7126, 98.2475) (52.8378, 98.7209) knots 0 0 0 1 2 2 2
  spline S132 degree 2 poles (52.8378, 98.7209) (52.5496, 98.8856) (51.5822, 99.2664) (50.975, 99.5134) knots 0 0 0 1 2 2 2
  spline S133 degree 2 poles (50.975, 99.5134) (50.2751, 99.0502) (49.5238, 97.6711) (49.5238, 96.7963) knots 0 0 0 1 2 2 2
  spline S134 degree 2 poles (49.5238, 96.7963) (49.5238, 95.6437) (50.9132, 94.1411) (51.963, 94.1411) knots 0 0 0 1 2 2 2
  spline S135 degree 2 poles (51.963, 94.1411) (53.0333, 94.1411) (54.3301, 95.4275) (54.3301, 96.5391) knots 0 0 0 1 2 2 2
  spline S136 degree 2 poles (54.0934, 102.8993) (54.0934, 103.7536) (52.951, 104.8959) (51.9321, 104.8959) knots 0 0 0 1 2 2 2
  spline S137 degree 2 poles (51.9321, 104.8959) (51.0058, 104.8959) (49.8223, 103.8771) (49.8223, 103.0023) knots 0 0 0 1 2 2 2
  spline S138 degree 2 poles (49.8223, 103.0023) (49.8223, 102.3745) (50.4295, 101.4997) (51.0367, 101.1498) knots 0 0 0 1 2 2 2
  spline S139 degree 2 poles (51.0367, 101.1498) (51.294, 101.0057) (52.3849, 100.5014) (52.8275, 100.3573) knots 0 0 0 1 2 2 2
  spline S140 degree 2 poles (52.8275, 100.3573) (53.5685, 100.9233) (54.0934, 102.1275) (54.0934, 102.8993) knots 0 0 0 1 2 2 2
  line L361 (59.5377, 106.4294) -> (59.1672, 101.4894)
  line L362 (59.1672, 101.4894) -> (58.0454, 101.4894)
  line L363 (58.0454, 101.4894) -> (57.6749, 106.4294)
  line L364 (57.6749, 106.4294) -> (59.5377, 106.4294)
  line L365 (62.7487, 106.4294) -> (62.3782, 101.4894)
  line L366 (62.3782, 101.4894) -> (61.2564, 101.4894)
  line L367 (61.2564, 101.4894) -> (60.8859, 106.4294)
  line L368 (60.8859, 106.4294) -> (62.7487, 106.4294)
  line L369 (67.9769, 95.5922) -> (65.5892, 90.0038)
  line L370 (65.5892, 90.0038) -> (64.3439, 90.0038)
  line L371 (64.3439, 90.0038) -> (65.8465, 95.5922)
  line L372 (65.8465, 95.5922) -> (67.9769, 95.5922)
  line L373 (77.1263, 93.1634) -> (70.9306, 93.1634)
  line L374 (70.9306, 93.1634) -> (70.9306, 94.4601)
  line L375 (70.9306, 94.4601) -> (73.236, 94.4601)
  line L376 (73.236, 94.4601) -> (73.236, 102.9714)
  line L377 (73.236, 102.9714) -> (70.9306, 102.9714)
  line L378 (70.9306, 102.9714) -> (70.9306, 104.1344)
  spline S141 degree 2 poles (70.9306, 104.1344) (72.2377, 104.1344) (73.4727, 104.8754) (73.555, 105.9045) knots 0 0 0 1 2 2 2
  line L379 (73.555, 105.9045) -> (74.8724, 105.9045)
  line L380 (74.8724, 105.9045) -> (74.8724, 94.4601)
  line L381 (74.8724, 94.4601) -> (77.1263, 94.4601)
  line L382 (77.1263, 94.4601) -> (77.1263, 93.1634)
  line L383 (84.7421, 106.4294) -> (79.7712, 90.4052)
  line L384 (79.7712, 90.4052) -> (78.3304, 90.4052)
  line L385 (78.3304, 90.4052) -> (83.2807, 106.4294)
  line L386 (83.2807, 106.4294) -> (84.7421, 106.4294)
  line L387 (93.9738, 93.1634) -> (86.1418, 93.1634)
  line L388 (86.1418, 93.1634) -> (86.1418, 94.9644)
  spline S142 degree 2 poles (86.1418, 94.9644) (86.9857, 95.7569) (88.4883, 97.2286) (89.2087, 98.0211) knots 0 0 0 1 2 2 2
  spline S143 degree 2 poles (89.2087, 98.0211) (90.6599, 99.6163) (91.7199, 101.5305) (91.7199, 102.5494) knots 0 0 0 1 2 2 2
  spline S144 degree 2 poles (91.7199, 102.5494) (91.7199, 103.0846) (91.3906, 103.8874) (91.0921, 104.1446) knots 0 0 0 1 2 2 2
  spline S145 degree 2 poles (91.0921, 104.1446) (90.7937, 104.4019) (90.0115, 104.6592) (89.5381, 104.6592) knots 0 0 0 1 2 2 2
  spline S146 degree 2 poles (89.5381, 104.6592) (89.0852, 104.6592) (88.159, 104.4328) (87.737, 104.2579) knots 0 0 0 1 2 2 2
  spline S147 degree 2 poles (87.737, 104.2579) (87.3768, 104.1138) (86.7079, 103.7021) (86.502, 103.558) knots 0 0 0 1 2 2 2
  line L389 (86.502, 103.558) -> (86.4094, 103.558)
  line L390 (86.4094, 103.558) -> (86.4094, 105.3694)
  spline S148 degree 2 poles (86.4094, 105.3694) (86.9343, 105.6267) (88.8177, 106.131) (89.6616, 106.131) knots 0 0 0 1 2 2 2
  spline S149 degree 2 poles (89.6616, 106.131) (91.4421, 106.131) (93.4489, 104.2476) (93.4489, 102.6421) knots 0 0 0 1 2 2 2
  spline S150 degree 2 poles (93.4489, 102.6421) (93.4489, 101.8908) (93.099, 100.6352) (92.7903, 100.1) knots 0 0 0 1 2 2 2
  spline S151 degree 2 poles (92.7903, 100.1) (92.4815, 99.5442) (91.5861, 98.4533) (91.0921, 97.9284) knots 0 0 0 1 2 2 2
  spline S152 degree 2 poles (91.0921, 97.9284) (90.2894, 97.0536) (88.3237, 95.1805) (87.737, 94.6351) knots 0 0 0 1 2 2 2
  line L391 (87.737, 94.6351) -> (93.9738, 94.6351)
  line L392 (93.9738, 94.6351) -> (93.9738, 93.1634)
  line L393 (97.5759, 106.4294) -> (97.2054, 101.4894)
  line L394 (97.2054, 101.4894) -> (96.0836, 101.4894)
  line L395 (96.0836, 101.4894) -> (95.7131, 106.4294)
  line L396 (95.7131, 106.4294) -> (97.5759, 106.4294)
  line L397 (100.7869, 106.4294) -> (100.4164, 101.4894)
  line L398 (100.4164, 101.4894) -> (99.2946, 101.4894)
  line L399 (99.2946, 101.4894) -> (98.9241, 106.4294)
  line L400 (98.9241, 106.4294) -> (100.7869, 106.4294)
  line L401 (106.0152, 95.5922) -> (103.6275, 90.0038)
  line L402 (103.6275, 90.0038) -> (102.3822, 90.0038)
  line L403 (102.3822, 90.0038) -> (103.8848, 95.5922)
  line L404 (103.8848, 95.5922) -> (106.0152, 95.5922)
  spline S153 degree 2 poles (111.3977, 104.6592) (110.9346, 104.6592) (110.0186, 104.4328) (109.5761, 104.2579) knots 0 0 0 1 2 2 2
  spline S154 degree 2 poles (109.5761, 104.2579) (109.1644, 104.0829) (108.5572, 103.7124) (108.3205, 103.5477) knots 0 0 0 1 2 2 2
  line L405 (108.3205, 103.5477) -> (108.2176, 103.5477)
  line L406 (108.2176, 103.5477) -> (108.2176, 105.3488)
  spline S155 degree 2 poles (108.2176, 105.3488) (108.7733, 105.6472) (110.6773, 106.131) (111.5315, 106.131) knots 0 0 0 1 2 2 2
  spline S156 degree 2 poles (111.5315, 106.131) (112.396, 106.131) (113.6825, 105.781) (114.2074, 105.4105) knots 0 0 0 1 2 2 2
  spline S157 degree 2 poles (114.2074, 105.4105) (114.7631, 105.0092) (115.3395, 103.8462) (115.3395, 103.064) knots 0 0 0 1 2 2 2
  spline S158 degree 2 poles (115.3395, 103.064) (115.3395, 102.0143) (113.9604, 100.4293) (112.9929, 100.2235) knots 0 0 0 1 2 2 2
  line L407 (112.9929, 100.2235) -> (112.9929, 100.1)
  spline S159 degree 2 poles (112.9929, 100.1) (113.3943, 100.0177) (114.3103, 99.6472) (114.7014, 99.2767) knots 0 0 0 1 2 2 2
  spline S160 degree 2 poles (114.7014, 99.2767) (115.0925, 98.9164) (115.5865, 97.7638) (115.5865, 96.9301) knots 0 0 0 1 2 2 2
  spline S161 degree 2 poles (115.5865, 96.9301) (115.5865, 96.0759) (114.9998, 94.6248) (114.4647, 94.069) knots 0 0 0 1 2 2 2
  spline S162 degree 2 poles (114.4647, 94.069) (113.9089, 93.4927) (112.3343, 92.8958) (111.336, 92.8958) knots 0 0 0 1 2 2 2
  spline S163 degree 2 poles (111.336, 92.8958) (110.3788, 92.8958) (108.5057, 93.3589) (107.8677, 93.678) knots 0 0 0 1 2 2 2
  line L408 (107.8677, 93.678) -> (107.8677, 95.479)
  line L409 (107.8677, 95.479) -> (107.9912, 95.479)
  spline S164 degree 2 poles (107.9912, 95.479) (108.5263, 95.0879) (110.3377, 94.3675) (111.2331, 94.3675) knots 0 0 0 1 2 2 2
  spline S165 degree 2 poles (111.2331, 94.3675) (111.7579, 94.3675) (112.8077, 94.6968) (113.1576, 95.0776) knots 0 0 0 1 2 2 2
  spline S166 degree 2 poles (113.1576, 95.0776) (113.4972, 95.4584) (113.8575, 96.3641) (113.8575, 97.0536) knots 0 0 0 1 2 2 2
  spline S167 degree 2 poles (113.8575, 97.0536) (113.8575, 97.7432) (113.4561, 98.6386) (113.0959, 98.8959) knots 0 0 0 1 2 2 2
  spline S168 degree 2 poles (113.0959, 98.8959) (112.7357, 99.1532) (111.7579, 99.3487) (111.1816, 99.3487) knots 0 0 0 1 2 2 2
  line L410 (111.1816, 99.3487) -> (110.4612, 99.3487)
  line L411 (110.4612, 99.3487) -> (110.4612, 100.7587)
  line L412 (110.4612, 100.7587) -> (111.0272, 100.7587)
  spline S169 degree 2 poles (111.0272, 100.7587) (112.1696, 100.7587) (113.6104, 101.8496) (113.6104, 102.8891) knots 0 0 0 1 2 2 2
  spline S170 degree 2 poles (113.6104, 102.8891) (113.6104, 103.3728) (113.2399, 104.0623) (112.9415, 104.2681) knots 0 0 0 1 2 2 2
  spline S171 degree 2 poles (112.9415, 104.2681) (112.6224, 104.4843) (111.8403, 104.6592) (111.3977, 104.6592) knots 0 0 0 1 2 2 2
  line L413 (122.7804, 106.4294) -> (117.8095, 90.4052)
  line L414 (117.8095, 90.4052) -> (116.3686, 90.4052)
  line L415 (116.3686, 90.4052) -> (121.319, 106.4294)
  line L416 (121.319, 106.4294) -> (122.7804, 106.4294)
  line L417 (132.3517, 97.5271) -> (130.8388, 97.5271)
  line L418 (130.8388, 97.5271) -> (130.8388, 93.1634)
  line L419 (130.8388, 93.1634) -> (129.2024, 93.1634)
  line L420 (129.2024, 93.1634) -> (129.2024, 97.5271)
  line L421 (129.2024, 97.5271) -> (123.5934, 97.5271)
  line L422 (123.5934, 97.5271) -> (123.5934, 99.3178)
  line L423 (123.5934, 99.3178) -> (129.2745, 105.8634)
  line L424 (129.2745, 105.8634) -> (130.8388, 105.8634)
  line L425 (130.8388, 105.8634) -> (130.8388, 98.8959)
  line L426 (130.8388, 98.8959) -> (132.3517, 98.8959)
  line L427 (132.3517, 98.8959) -> (132.3517, 97.5271)
  line L428 (129.2024, 98.8959) -> (129.2024, 103.8565)
  line L429 (129.2024, 103.8565) -> (124.9314, 98.8959)
  line L430 (124.9314, 98.8959) -> (129.2024, 98.8959)
  line L431 (138.8252, 106.4294) -> (138.4547, 101.4894)
  line L432 (138.4547, 101.4894) -> (137.3329, 101.4894)
  line L433 (137.3329, 101.4894) -> (136.9624, 106.4294)
  line L434 (136.9624, 106.4294) -> (138.8252, 106.4294)
  line L435 (135.6142, 106.4294) -> (135.2437, 101.4894)
  line L436 (135.2437, 101.4894) -> (134.1219, 101.4894)
  line L437 (134.1219, 101.4894) -> (133.7514, 106.4294)
  line L438 (133.7514, 106.4294) -> (135.6142, 106.4294)
  spline S172 degree 2 poles (145.5663, 98.0416) (145.5663, 95.407) (143.8784, 91.4138) (142.3861, 89.6539) knots 0 0 0 1 2 2 2
  line L439 (142.3861, 89.6539) -> (140.4307, 89.6539)
  line L440 (140.4307, 89.6539) -> (140.4307, 89.7362)
  spline S173 degree 2 poles (140.4307, 89.7362) (141.0894, 90.3228) (142.417, 92.0416) (142.911, 93.0707) knots 0 0 0 1 2 2 2
  spline S174 degree 2 poles (142.911, 93.0707) (143.4462, 94.172) (144.0637, 96.6214) (144.0637, 98.0416) knots 0 0 0 1 2 2 2
  spline S175 degree 2 poles (144.0637, 98.0416) (144.0637, 99.4516) (143.4359, 101.9525) (142.911, 103.0126) knots 0 0 0 1 2 2 2
  spline S176 degree 2 poles (142.911, 103.0126) (142.3964, 104.0726) (141.0791, 105.7604) (140.4307, 106.3471) knots 0 0 0 1 2 2 2
  line L441 (140.4307, 106.3471) -> (140.4307, 106.4294)
  line L442 (140.4307, 106.4294) -> (142.3861, 106.4294)
  spline S177 degree 2 poles (142.3861, 106.4294) (143.8681, 104.6695) (145.5663, 100.6969) (145.5663, 98.0416) knots 0 0 0 1 2 2 2
  line L443 (-140.4719, 77.0388) -> (-145.2781, 77.0388)
  line L444 (-145.2781, 77.0388) -> (-145.2781, 78.5826)
  line L445 (-145.2781, 78.5826) -> (-140.4719, 78.5826)
  line L446 (-140.4719, 78.5826) -> (-140.4719, 77.0388)
  line L447 (-125.6106, 72.2532) -> (-132.9692, 72.2532)
  line L448 (-132.9692, 72.2532) -> (-132.9692, 84.9532)
  line L449 (-132.9692, 84.9532) -> (-131.2814, 84.9532)
  line L450 (-131.2814, 84.9532) -> (-131.2814, 73.7557)
  line L451 (-131.2814, 73.7557) -> (-125.6106, 73.7557)
  line L452 (-125.6106, 73.7557) -> (-125.6106, 72.2532)
  spline S178 degree 2 poles (-120.2692, 72.037) (-122.554, 72.037) (-125.0652, 74.5997) (-125.0652, 76.9668) knots 0 0 0 1 2 2 2
  spline S179 degree 2 poles (-125.0652, 76.9668) (-125.0652, 79.2927) (-122.626, 82.0509) (-120.6603, 82.0509) knots 0 0 0 1 2 2 2
  spline S180 degree 2 poles (-120.6603, 82.0509) (-119.7752, 82.0509) (-118.4064, 81.5363) (-117.9021, 80.9908) knots 0 0 0 1 2 2 2
  spline S181 degree 2 poles (-117.9021, 80.9908) (-117.3875, 80.4454) (-116.8421, 78.8707) (-116.8421, 77.7284) knots 0 0 0 1 2 2 2
  line L453 (-116.8421, 77.7284) -> (-116.8421, 76.8536)
  line L454 (-116.8421, 76.8536) -> (-123.4391, 76.8536)